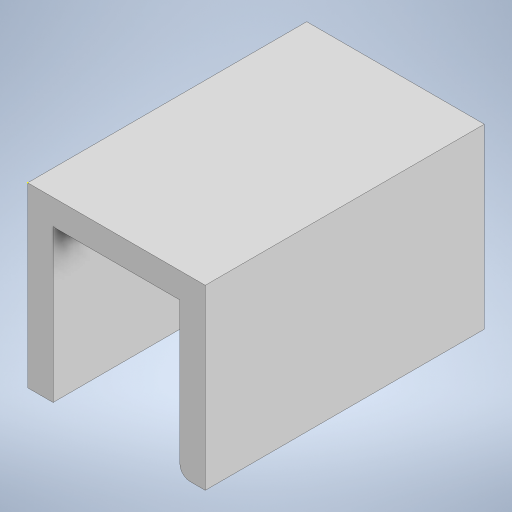
# Autodesk Inventor part: housing_v07
Saved by Autodesk Inventor 2023 (Build 270158000, 158)
## iProperties
Created: 2023-11-20
Part Number: housing_v07
Material: Generic
Document SubType Name: Modeling
Designer: Akramilab
Density: 1 g/cm^3
Appearance: Default
Author: Akramilab
Autodesk Inventor part; units mm, degrees
ref_plane "YZ Plane" through (0, 0, 0) normal (1, 0, 0) x (0, 1, 0)
ref_plane "XZ Plane" through (0, 0, 0) normal (0, 1, 0) x (-1, 0, 0)
ref_plane "XY Plane" through (0, 0, 0) normal (0, 0, 1) x (1, 0, 0)
sketch "Sketch1" plane through (0, 0, 0) normal (0, 0, 1) x (1, 0, 0)
  line L0 (0, 0) -> (14, 0)
  line L1 (14, 0) -> (14, -14)
  line L2 (14, -14) -> (0, -14)
  line L3 (0, -14) -> (0, 0)
  dimension "d0" = 14
  dimension "d1" = 14
  constraints: 8 end point, 2 parallel, 1 horizontal, 1 perpendicular
  measures "d0" distance of L1.end L2.end
  measures "d1" distance of L0.end L1.end
extrude "Extrusion1" add sketch "Sketch1" against normal blind 22
sketch "Sketch2" plane through (0, 0, 0) normal (0, 0, 1) x (1, 0, 0)
  line L0 (2, -2) -> (12, -2)
  line L1 (12, -2) -> (12, -22)
  line L2 (12, -22) -> (2, -22)
  line L3 (2, -22) -> (2, -2)
  point P0 (0, 0)
  dimension "d4" = 10
  dimension "d5" = 20
  constraints: 8 end point, 2 parallel, 1 horizontal, 1 perpendicular
  measures "d4" distance of L1.end L2.end
  measures "d5" distance of L0.end L1.end
extrude "Extrusion2" cut sketch "Sketch2" against normal blind 20
sketch "Sketch8" plane through (0, -14, 0) normal (-1, 0, 0) x (0, 0, 1)
  point P0 (0, 14)
sketch "Sketch9" plane through (0, -14, 0) normal (-1, 0, 0) x (0, 0, 1)
  point P0 (0, 14)
sketch "Sketch11" plane through (0, -14, 0) normal (-1, 0, 0) x (0, 0, 1)
  point P0 (0, 14)
sketch "Sketch14" plane through (0, -14, 0) normal (-1, 0, 0) x (0, 0, 1)
  point P0 (0, 14)
sketch "Sketch15" plane through (0, -14, 0) normal (-1, 0, 0) x (0, 0, 1)
  point P0 (0, 14)
sketch "Sketch16" plane through (0, -14, 0) normal (-1, 0, 0) x (0, 0, 1)
  line L0 (-12.5, 12) -> (-17.5, 12)
  line L1 (-17.5, 12) -> (-17.5, 0)
  line L2 (-17.5, 0) -> (-12.5, 0)
  line L3 (-12.5, 0) -> (-12.5, 12)
  point P0 (0, 14)
  dimension "d30" = 5
  dimension "d31" = 12
  constraints: 8 end point, 2 parallel, 1 horizontal, 1 perpendicular
  measures "d30" distance of L2.end L1.end
  measures "d31" distance of L1.end L0.end
extrude "Extrusion10" cut sketch "Sketch16" against normal blind 2
sketch "Sketch17" plane through (0, 0, -20) normal (0, 0, 1) x (1, 0, 0)
  line L0 (12, -2) -> (7.5, -2)
  line L1 (7.5, -2) -> (7.5, -6.5)
  line L2 (7.5, -6.5) -> (12, -6.5)
  line L3 (12, -6.5) -> (12, -2)
  point P0 (0, 0)
  dimension "d34" = 4.5
  dimension "d35" = 4.5
  constraints: 8 end point, 2 parallel, 1 horizontal, 1 perpendicular
  measures "d34" distance of L2.end L1.end
  measures "d35" distance of L1.end L0.end
extrude "Extrusion11" add sketch "Sketch17" along normal blind 9
fillet "Fillet1" radius 0.8 8 edges at (0, -8, -12.5) (2, -8, -12.5) (0, -2, -15) (0, -8, -17.5) (2, -8, -17.5) (12, -14, -10) (7.5, -6.5, -15.5) (9.75, -6.5, -11)
body "Solid1"
